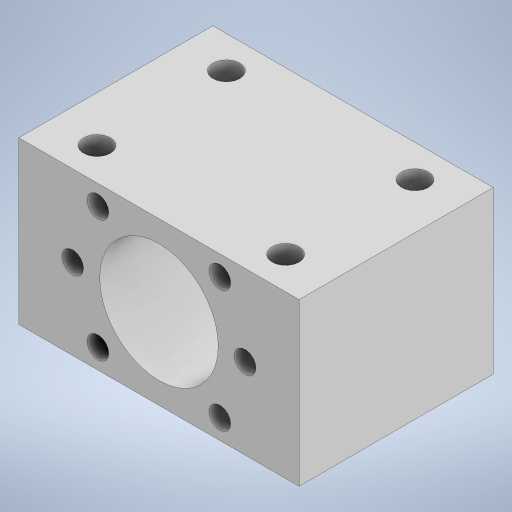
# Autodesk Inventor part: DSG16H
Saved by Autodesk Inventor 2023 (Build 270158000, 158)
## iProperties
Created: 2022-05-01
Part Number: DSG16H
Material: Generic
Document SubType Name: Modeling
Designer: plebbb
Density: 1 g/cm^3
Appearance: Default
Author: plebbb
Autodesk Inventor part; units mm, degrees
ref_plane "YZ Plane" through (0, 0, 0) normal (1, 0, 0) x (0, 1, 0)
ref_plane "XZ Plane" through (0, 0, 0) normal (0, 1, 0) x (-1, 0, 0)
ref_plane "XY Plane" through (0, 0, 0) normal (0, 0, 1) x (1, 0, 0)
sketch "Sketch1" plane through (0, 0, 0) normal (0, 0, 1) x (1, 0, 0)
  circle A0 centre (0, 0) radius 11
  line L0 (-26, -15) -> (26, -15)
  line L1 (26, -15) -> (26, 15)
  line L2 (-26, 15) -> (-26, -15)
  circle A1 centre (0, 0) radius 16 construction
  circle A2 centre (11.3137, 11.3137) radius 2
  circle A3 centre (-11.3137, -11.3137) radius 2
  circle A4 centre (11.3137, -11.3137) radius 2
  circle A5 centre (-11.3137, 11.3137) radius 2
  circle A6 centre (-16, 0) radius 2
  circle A7 centre (16, 0) radius 2
  line L3 (-11.3137, 11.3137) -> (0, 0) construction
  line L4 (0, 0) -> (-16, 0) construction
  line L5 (-26, 15) -> (26, 15)
  point P0 (0, -15)
  dimension "d0" = 22
  dimension "d2" = 52
  dimension "d3" = 32
  dimension "d4" = 4
  dimension "d5" = 45
  dimension "d6" = 15
  dimension "d16" = 30
  constraints: 12 end point, 8 centre point, 6 point on circle, 5 equal radius, 3 horizontal, 3 horizontal alignment, 3 vertical alignment, 2 coincident, 2 perpendicular, 1 midpoint, 1 parallel
  measures "d0" diameter of A0
  measures "d2" distance of L0.start L0.end
  measures "d3" diameter of A1
  measures "d4" diameter of A5
  measures "d5" angle of L3 L4
  measures "d6" distance from line of L0 A0.centre
  measures "d16" distance of L0.end L1.end
extrude "Extrusion1" add sketch "Sketch1" along normal blind 36
sketch "Sketch3" plane through (-26, 15, 0) normal (0, 1, 0) x (1, 0, 0)
  circle A0 centre (8.5, -6) radius 2.5
  circle A1 centre (43.5, -6) radius 2.5
  circle A2 centre (43.5, -30) radius 2.5
  circle A3 centre (8.5, -30) radius 2.5
  line L0 (8.5, -6) -> (43.5, -6) construction
  line L1 (43.5, -6) -> (43.5, -30) construction
  line L2 (43.5, -30) -> (8.5, -30) construction
  line L3 (8.5, -30) -> (8.5, -6) construction
  line L4 (52, 0) -> (0, 0) construction
  line L5 (52, 0) -> (52, -36) construction
  point P0 (26, 0)
  point P1 (26, -6)
  point P2 (26, 0)
  point P3 (43.5, -18)
  point P4 (52, -18)
  dimension "d17" = 5
  dimension "d18" = 35
  dimension "d19" = 24
  constraints: 8 end point, 4 centre point, 4 coincident, 4 midpoint, 3 equal radius, 2 parallel, 1 horizontal, 1 horizontal alignment, 1 perpendicular, 1 vertical alignment
  measures "d17" diameter of A1
  measures "d18" distance of L0.start L0.end
  measures "d19" distance of L0.end L1.end
extrude "Extrusion3" cut sketch "Sketch3" against normal blind 10
body "Solid1"
